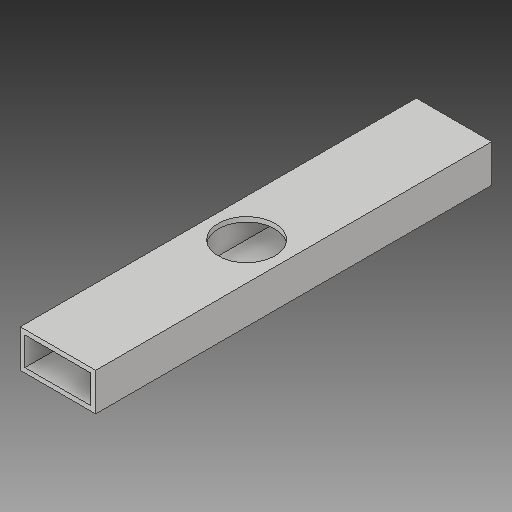
# Autodesk Inventor part: Motor Mount
Saved by Autodesk Inventor 2018 (Build 220112000, 112)
## iProperties
Created: 2018-01-29
Part Number: Motor Mount
Material: Generic
Document SubType Name: Modeling
Designer: Apple
Density: 1 g/cm^3
Appearance: Default
Author: Apple
Autodesk Inventor part; units mm, degrees
ref_plane "YZ Plane" through (0, 0, 0) normal (1, 0, 0) x (0, 1, 0)
ref_plane "XZ Plane" through (0, 0, 0) normal (0, 1, 0) x (-1, 0, 0)
ref_plane "XY Plane" through (0, 0, 0) normal (0, 0, 1) x (1, 0, 0)
sketch "Sketch1" plane through (0, 0, 0) normal (0, 0, 1) x (1, 0, 0)
  line L0 (37.2518, 31.5045) -> (-13.5482, 31.5045)
  line L1 (-13.5482, 31.5045) -> (-13.5482, 6.1045)
  line L2 (-13.5482, 6.1045) -> (37.2518, 6.1045)
  line L3 (37.2518, 6.1045) -> (37.2518, 31.5045)
  line L4 (34.0768, 28.3295) -> (-10.3732, 28.3295)
  line L5 (-10.3732, 28.3295) -> (-10.3732, 9.2795)
  line L6 (-10.3732, 9.2795) -> (34.0768, 9.2795)
  line L7 (34.0768, 9.2795) -> (34.0768, 28.3295)
  point P0 (0, 0)
  dimension "d0" = 50.8
  dimension "d1" = 25.4
  dimension "d2" = 3.175
  constraints: 16 end point, 4 parallel, 2 perpendicular, 1 horizontal, 3 other
  measures "d0" distance of L0.start L0.end
  measures "d1" distance of L2.end L0.start
  measures "d2" distance between parallel lines of L3 L7
extrude "Extrusion1" add sketch "Sketch1" against normal blind 177.8 and the other way blind 88.9
sketch "Sketch2" plane through (-13.5482, 31.5045, -177.8) normal (0, 1, 0) x (1, 0, 0)
  circle A0 centre (25.4, -139.7) radius 19.05
  line L0 (50.8, -266.7) -> (0, -266.7) projected
  point P0 (13.5482, -177.8)
  point P1 (25.4, -266.7)
  dimension "d7" = 38.1
  dimension "d8" = 127
  constraints: 1 centre point, 1 midpoint, 1 vertical alignment
  measures "d7" diameter of A0
  measures "d8" distance from line of A0.centre L0
extrude "Extrusion2" cut sketch "Sketch2" against normal blind 3.175
body "Solid1"
